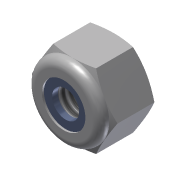
# Autodesk Inventor part: 8-32 locknut
Saved by Autodesk Inventor 2013 (Build 170138000, 138)
## iProperties
Created: 2012-12-09
Part Number: 8-32 locknut
Material: Steel
Document SubType Name: Modeling
Designer: Nemo
Density: 1 g/cm^3
Author: Nemo
Autodesk Inventor part; units mm, degrees
ref_plane "YZ Plane" through (0, 0, 0) normal (1, 0, 0) x (0, 1, 0)
ref_plane "XZ Plane" through (0, 0, 0) normal (0, 1, 0) x (-1, 0, 0)
ref_plane "XY Plane" through (0, 0, 0) normal (0, 0, 1) x (1, 0, 0)
sketch "Sketch1" plane through (0, 0, 0) normal (0, 0, 1) x (1, 0, 0)
  line L0 (-2.5205, 4.3656) -> (2.5205, 4.3656)
  line L1 (2.5205, 4.3656) -> (5.041, 0)
  line L2 (5.041, 0) -> (2.5205, -4.3656)
  line L3 (2.5205, -4.3656) -> (-2.5205, -4.3656)
  line L4 (-2.5205, -4.3656) -> (-5.041, 0)
  line L5 (-5.041, 0) -> (-2.5205, 4.3656)
  point P0 (0, 0)
  point P1 (0, 0)
  dimension "d0" = 8.7312
  constraints: 12 end point, 1 coincident, 1 horizontal, 13 other
  measures "d0" distance between parallel lines of L0 L3
extrude "Extrusion1" add sketch "Sketch1" along normal blind 4.953
sketch "Sketch2" plane through (0, 0, 0) normal (1, 0, 0) x (0, 1, 0)
  line L0 (4.3656, 4.953) -> (4.3656, 0) construction
  line L1 (4.3656, 0) -> (-4.3656, 0) construction
  line L2 (-4.3656, 0) -> (-4.3656, 4.953) construction
  line L3 (-4.3656, 4.953) -> (4.3656, 4.953) construction
  line L4 (0, 4.953) -> (0, 5.9436)
  line L5 (-4.3656, 4.953) -> (0, 4.953)
  arc A0 (-3.3782, 5.9436) -> (-4.3688, 4.953) centre (-3.3782, 4.953) ccw
  line L6 (-3.3782, 5.9436) -> (0, 5.9436)
  line L7 (0, 5.9436) -> (0, 4.953)
  line L8 (0, 4.953) -> (-4.3688, 4.953)
  point P0 (0, 0)
  dimension "d6" = 0.9906
  dimension "d7" = 3.3782
  constraints: 10 end point, 3 perpendicular, 2 point on circle, 1 centre point, 1 collinear, 1 midpoint, 1 parallel, 1 point on line, 1 tangent
  measures "d6" radius of A0
  measures "d7" distance of L4.start A0.centre
revolve "Revolution1" add sketch "Sketch2" angle 360 about axis through (0, 0, 4.953) along (0, 0, 1)
sketch "Sketch3" plane through (0, 0, 0) normal (0, 1, 0) x (-1, 0, 0)
  arc A0 (-3.3782, 5.9436) -> (-4.3688, 4.953) centre (-3.3782, 4.953) ccw construction
  line L0 (-3.3782, 5.9436) -> (3.3782, 5.9436) construction
  arc A1 (4.3688, 4.953) -> (3.3782, 5.9436) centre (3.3782, 4.953) ccw construction
  line L1 (4.3688, 4.953) -> (5.041, 4.953) construction
  line L2 (5.041, 4.953) -> (5.041, 0) construction
  line L3 (5.041, 0) -> (-5.041, 0) construction
  line L4 (-5.041, 0) -> (-5.041, 4.953) construction
  line L5 (-5.041, 4.953) -> (-4.3688, 4.953) construction
  line L6 (-4.3552, 4.953) -> (-5.041, 4.6482)
  line L7 (-5.041, 4.6482) -> (-5.041, 4.953)
  line L8 (-5.041, 4.953) -> (-4.3552, 4.953)
  line L9 (0, 0) -> (0, 7.4764) construction
  line L10 (-5.041, 0.3048) -> (-4.3552, 0)
  line L11 (-5.041, 0.3048) -> (-5.041, 0)
  line L12 (-5.041, 0) -> (-4.3552, 0)
  dimension "d9" = 0.6858
  dimension "d10" = 0.3048
  dimension "d11" = 0.3048
  dimension "d12" = 0.6858
  constraints: 14 end point, 4 point on line, 3 collinear, 2 perpendicular
  measures "d9" distance of L4.end L6.start
  measures "d10" distance of L4.end L6.end
  measures "d11" distance of L3.end L10.start
  measures "d12" distance of L3.end L10.end
revolve "Revolution2" cut sketch "Sketch3" angle 360 about axis through (0, 0, 0) along (0, 0, 1)
sketch "Sketch4" plane through (0, 0, 5.9436) normal (0, 0, 1) x (1, 0, 0)
  circle A0 centre (0, 0) radius 3.3782 projected
hole "Hole1" at (0, 0, 5.9436) direction (0, 0, -1) diameter 3.302 end through all counterbore diameter 5.1054 counterbore depth 0.2286 thread size "8-32 UNC" class "2B" standard "ANSI Unified Screw Threads"
sketch "Sketch5" plane through (0, 0, 5.715) normal (0, 0, 1) x (1, 0, 0)
  circle A0 centre (0, 0) radius 1.651 projected
  circle A1 centre (0, 0) radius 1.5875
  dimension "d21" = 3.175
  constraints: 1 centre point, 1 coincident
  measures "d21" diameter of A1
extrude "Extrusion2" add sketch "Sketch5" against normal blind 0.6858
equation "\"d6\" = d5"
equation "\"d5\" = 0.9906"
body "Solid1"
